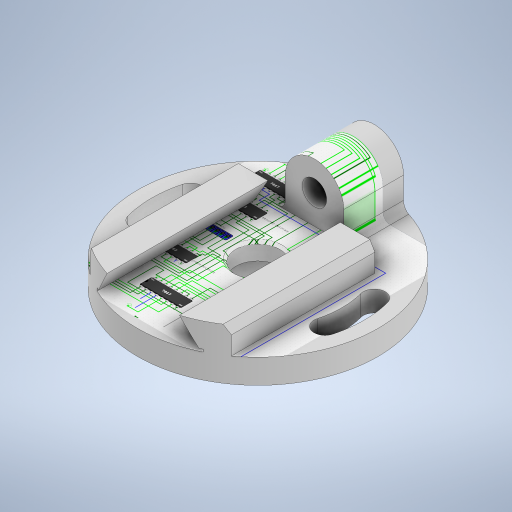
# Autodesk Inventor part: 05-16-2023 Piattaforma
Saved by Autodesk Inventor 2023 (Build 270158000, 158)
## iProperties
Created: 2023-05-16
Part Number: 05-16-2023 Piattaforma
Material: Generico
Document SubType Name: Modeling
Designer: Admin
Density: 1 g/cm^3
Appearance: Default
Author: Admin
Autodesk Inventor part; units mm, degrees
ref_plane "YZ Plane" through (0, 0, 0) normal (1, 0, 0) x (0, 1, 0)
ref_plane "XZ Plane" through (0, 0, 0) normal (0, 1, 0) x (-1, 0, 0)
ref_plane "XY Plane" through (0, 0, 0) normal (0, 0, 1) x (1, 0, 0)
sketch "Schizzo1" plane through (0, 0, 0) normal (0, 0, 1) x (1, 0, 0)
  line L0 (0, 0) -> (0, 364.6475) construction
  line L1 (44, 0) -> (44, 25)
  line L2 (44, 25) -> (92.5, 25)
  line L3 (92.5, 25) -> (92.5, 22)
  line L4 (92.5, 22) -> (98.5, 22)
  line L5 (98.5, 22) -> (98.5, 42)
  line L6 (98.5, 42) -> (58, 42)
  line L7 (58, 42) -> (58, 64)
  line L8 (58, 64) -> (29.6906, 64)
  line L9 (29.6906, 64) -> (41.2376, 44)
  line L10 (41.2376, 44) -> (43.5, 44)
  line L11 (43.5, 44) -> (43.5, 42)
  line L12 (43.5, 42) -> (18, 42)
  line L13 (18, 42) -> (18, 28)
  line L14 (18, 28) -> (33.5, 28)
  line L15 (33.5, 28) -> (33.5, 25)
  line L16 (33.5, 25) -> (29, 25)
  line L17 (29, 25) -> (29, 0)
  line L18 (29, 0) -> (44, 0)
  line L19 (43.5, 42) -> (58, 42)
  circle A0 centre (32, 48) radius 6 construction
  line L20 (58, 58.7181) -> (65, 58.7181) construction
  dimension "d0" = 197
  dimension "d1" = 185
  dimension "d2" = 116
  dimension "d3" = 88
  dimension "d4" = 67
  dimension "d5" = 58
  dimension "d6" = 87
  dimension "d7" = 36
  dimension "d8" = 12
  dimension "d9" = 64
  dimension "d10" = 22
  dimension "d11" = 30
  dimension "d12" = 20
  dimension "d13" = 3
  dimension "d14" = 2
  dimension "d15" = 3
  dimension "d16" = 25
  constraints: 42 end point, 14 perpendicular, 3 point on line, 2 horizontal alignment, 2 parallel, 2 tangent, 2 vertical, 1 centre point, 1 horizontal
  measures "d0" diameter of L5 L0
  measures "d1" diameter of L3 L0
  measures "d2" diameter of L7 L0
  measures "d3" diameter of L1 L0
  measures "d4" diameter of L15 L0
  measures "d5" diameter of L17 L0
  measures "d6" diameter of L11 L0
  measures "d7" diameter of L13 L0
  measures "d8" diameter of A0
  measures "d9" diameter of A0.centre L0
  measures "d10" distance of L6.end L7.end
  measures "d11" angle of L0 L9
  measures "d12" distance of L4.end L5.end
  measures "d13" distance of L2.end L3.end
  measures "d14" distance of L10.end L11.end
  measures "d15" distance of L14.end L15.end
  measures "d16" distance of L1.start L1.end
revolve "Rivoluzione1" add sketch "Schizzo1" angle 360 about axis through (0, 0, 0) along (0, 1, 0) contours L18 L17 L16 L15 L14 L13 L12 L19 L6 L5 L4 L3 L2 L1
extrude "Estrusione1" add sketch "Schizzo1" along normal up to surface contours L19 L11 L10 L9 L8 L7 round surface about axis through (0, 32, 0) along (0, 1, 0) radius 98.5 far side no
extrude "Estrusione2" add sketch "Schizzo1" against normal blind 38 contours L19 L11 L10 L9 L8 L7
mirror "Specchio1" about plane through (0, 0, 0) normal (1, 0, 0) of "Estrusione2", "Estrusione1"
sketch "Schizzo2" plane through (0, 0, 0) normal (0, 0, 1) x (1, 0, 0)
  circle A0 centre (0, 66) radius 24
  line L0 (98.5, 42) -> (-98.5, 42) construction
  circle A1 centre (0, 66) radius 10
  line L1 (-24, 66) -> (24, 66) construction
  line L2 (-24, 66) -> (-24, 42)
  line L3 (24, 66) -> (24, 42)
  line L4 (-24, 42) -> (0, 42)
  line L5 (24, 42) -> (0, 42)
  line L6 (0, 0) -> (0, 135.2762) construction
  point P0 (58, 42)
  point P1 (-58, 42)
  dimension "d24" = 48
  dimension "d25" = 20
  dimension "d26" = 24
  constraints: 12 end point, 2 centre point, 2 perpendicular, 2 point on circle, 2 point on line, 1 coincident, 1 collinear, 1 horizontal, 1 midpoint, 1 tangent, 1 vertical, 1 other
  measures "d24" diameter of A0
  measures "d25" diameter of A1
  measures "d26" distance between parallel lines of L1 L0
extrude "Estrusione3" add sketch "Schizzo2" against normal up to surface round surface about axis through (0, 32, 0) along (0, 1, 0) radius 98.5 far side no
extrude "Estrusione4" cut sketch "Schizzo2" against normal blind 46.5
sketch "Schizzo3" plane through (43.5, 42, -38) normal (0, 1, 0) x (1, 0, 0)
  circle A0 centre (-43.5, -38) radius 18 construction
  circle A1 centre (-43.5, -38) radius 78 construction
  line L0 (14.5, 0) -> (14.5, -117.6131) construction
  line L1 (-101.5, 0) -> (-101.5, -117.6131) construction
  arc A2 (31.8422, -58.1879) -> (31.8422, -17.8121) centre (-43.5, -38) ccw construction
  arc A3 (40.5355, -60.5173) -> (40.5355, -15.4827) centre (-43.5, -38) ccw
  arc A4 (23.1489, -55.8585) -> (23.1489, -20.1415) centre (-43.5, -38) ccw
  arc A5 (23.1489, -55.8585) -> (40.5355, -60.5173) centre (31.8422, -58.1879) ccw
  arc A6 (40.5355, -15.4827) -> (23.1489, -20.1415) centre (31.8422, -17.8121) ccw
  line L2 (-43.5, -38) -> (-43.5, 58.5417) construction
  arc A7 (-127.5355, -15.4827) -> (-127.5355, -60.5173) centre (-43.5, -38) ccw
  arc A8 (-110.1489, -20.1415) -> (-110.1489, -55.8585) centre (-43.5, -38) ccw
  arc A9 (-127.5355, -60.5173) -> (-110.1489, -55.8585) centre (-118.8422, -58.1879) ccw
  arc A10 (-110.1489, -20.1415) -> (-127.5355, -15.4827) centre (-118.8422, -17.8121) ccw
  circle A11 centre (-43.5, -38) radius 98.5 projected
  line L3 (-67.5, 57.5314) -> (-19.5, 57.5314)
  point P0 (43.5, -38)
  dimension "d31" = 156
  dimension "d32" = 18
  dimension "d33" = 30
  dimension "d35" = 48
  constraints: 21 point on circle, 9 centre point, 6 symmetric about line, 4 end point, 4 tangent, 2 coincident, 1 horizontal, 1 horizontal alignment, 1 vertical, 8 other
  measures "d32" diameter of A5
  measures "d35" distance of L3.start L3.end
extrude "Estrusione5" cut sketch "Schizzo3" along normal blind 50.5 and the other way blind 23.25 contours A5 A4 A6 A3 | A10 A8 A9 A7 | L3 A11 picked at (-43.5, 58.5209)
fillet "Raccordo1" radius 6 3 edges at (24, 42, -71.0157) (-24, 42, -71.0157) (-44, 25, 0)
chamfer "Smusso1" distance 2 angle 45 3 edges at (-44, 0, 0) (-29, 0, 0) (-18, 42, 0)
chamfer "Smusso2" distance 7 angle 30 1 edges at (-58, 64, 20.8066) measured on face at (-58, 63.5, 20.8066)
chamfer "Smusso3" distance 7 angle 30 1 edges at (58, 64, 20.8066) measured on face at (58, 63.5, 20.8066)
sketch "Schizzo5" plane through (43.5, 42, -38) normal (0, 1, 0) x (1, 0, 0)
  line L0 (-118.1411, 40.7897) -> (36.6007, 40.7897) construction
  line L1 (36.6007, 40.7897) -> (36.6007, -129.405) construction
  line L2 (36.6007, -129.405) -> (-118.1411, -129.405) construction
  line L3 (-118.1411, -129.405) -> (-118.1411, 40.7897) construction
  point P0 (-43.5, -38)
  constraints: 2 other
decal "Decalcomania1"
